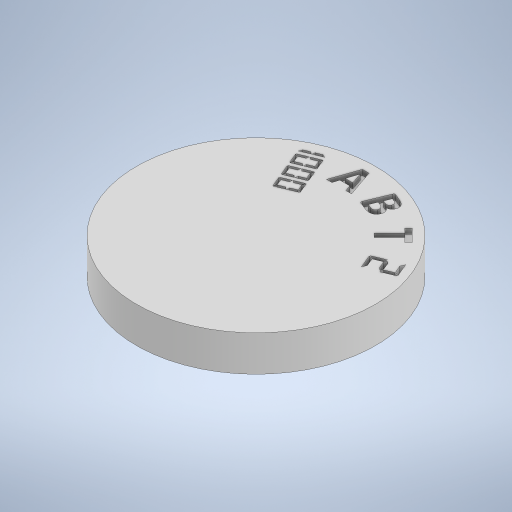
# Autodesk Inventor part: rot_th
Saved by Autodesk Inventor 2023 (Build 270158000, 158)
## iProperties
Created: 2023-05-20
Part Number: rot_th
Material: 常规
Document SubType Name: Modeling
Designer: LiuZeshu
Density: 1 g/cm^3
Appearance: 默认
Author: LiuZeshu
Autodesk Inventor part; units mm, degrees
ref_plane "YZ Plane" through (0, 0, 0) normal (1, 0, 0) x (0, 1, 0)
ref_plane "XZ Plane" through (0, 0, 0) normal (0, 1, 0) x (-1, 0, 0)
ref_plane "XY Plane" through (0, 0, 0) normal (0, 0, 1) x (1, 0, 0)
sketch "草图1" plane through (0, 0, 0) normal (0, 1, 0) x (-1, 0, 0)
  arc A0 (1.3748, -0.6) -> (-1.3748, -0.6) centre (0, 0) ccw
  line L0 (1.3748, -0.6) -> (-1.3748, -0.6)
  circle A1 centre (0, 0) radius 9
  dimension "d0" = 3
  dimension "d1" = 2.1
  dimension "d2" = 18
  constraints: 2 centre point, 2 coincident, 2 end point, 2 point on circle, 1 horizontal
  measures "d0" diameter of A0
  measures "d2" diameter of A1
extrude "拉伸1" add sketch "草图1" along normal blind 2.3
sketch "草图2" plane through (0, 2.3, 0) normal (0, 1, 0) x (1, 0, 0)
  circle A0 centre (0, 0) radius 9
  dimension "d7" = 18
  constraints: 1 centre point, 1 coincident
  measures "d7" diameter of A0
extrude "拉伸2" add sketch "草图2" along normal blind 0.4
sketch "草图3" plane through (0, 2.7, 0) normal (0, 1, 0) x (1, 0, 0)
  line L0 (0, 0) -> (0, 10.4823)
  line L1 (-0.7481, 7.9877) -> (0.7481, 7.9877) construction
  line L2 (0.7481, 7.9877) -> (0.7481, 6.3) construction
  line L3 (0.7481, 6.3) -> (-0.7481, 6.3) construction
  line L4 (-0.7481, 6.3) -> (-0.7481, 7.9877) construction
  line L5 (0, 0) -> (-4.0114, 9.6844)
  line L6 (0, 0) -> (-7.4121, 7.4121)
  line L7 (0, 0) -> (-9.6844, 4.0114)
  line L8 (0, 0) -> (-10.4823, 0)
  line L9 (0, 0) -> (-9.6844, -4.0114)
  line L10 (0, 0) -> (-7.4121, -7.4121)
  line L11 (0, 0) -> (-4.0114, -9.6844)
  line L12 (0, 0) -> (0, -10.4823)
  line L13 (0, 0) -> (4.0114, -9.6844)
  line L14 (0, 0) -> (7.4121, -7.4121)
  line L15 (0, 0) -> (9.6844, -4.0114)
  line L16 (0, 0) -> (10.4823, 0)
  line L17 (0, 0) -> (9.6844, 4.0114)
  line L18 (0, 0) -> (7.4121, 7.4121)
  line L19 (0, 0) -> (4.0114, 9.6844)
  line L20 (2.0839, 8.406) -> (4.4704, 7.4175) construction
  line L21 (4.4704, 7.4175) -> (3.6042, 5.3262) construction
  line L22 (3.6042, 5.3262) -> (1.2176, 6.3147) construction
  line L23 (1.2176, 6.3147) -> (2.0839, 8.406) construction
  line L24 (3.5415, 5.3681) -> (4.5678, 6.3944) construction
  line L25 (4.5678, 6.3944) -> (6.3944, 4.5678) construction
  line L26 (6.3944, 4.5678) -> (5.3681, 3.5415) construction
  line L27 (5.3681, 3.5415) -> (3.5415, 5.3681) construction
  line L28 (5.3262, 3.6042) -> (6.9301, 4.2685) construction
  line L29 (6.9301, 4.2685) -> (7.9186, 1.882) construction
  line L30 (7.9186, 1.882) -> (6.3147, 1.2176) construction
  line L31 (6.3147, 1.2176) -> (5.3262, 3.6042) construction
  line L32 (-4.0975, 7.4844) -> (-2.3949, 8.1897) construction
  line L33 (-2.3949, 8.1897) -> (-1.0621, 4.972) construction
  line L34 (-1.0621, 4.972) -> (-2.7647, 4.2668) construction
  line L35 (-2.7647, 4.2668) -> (-4.0975, 7.4844) construction
  line L36 (0.9024, 6.3013) -> (0.4624, 6.3013)
  line L37 (0.4624, 6.3013) -> (0.3119, 6.7554)
  line L38 (0.3119, 6.7554) -> (-0.4394, 6.7554)
  line L39 (-0.4394, 6.7554) -> (-0.5848, 6.3013)
  line L40 (-0.5848, 6.3013) -> (-0.9917, 6.3013)
  line L41 (-0.9917, 6.3013) -> (-0.2953, 8.3089)
  line L42 (-0.2953, 8.3089) -> (0.2034, 8.3089)
  line L43 (0.2034, 8.3089) -> (0.9024, 6.3013)
  line L44 (-0.0657, 7.9173) -> (-0.067, 7.9173)
  line L45 (-0.067, 7.9173) -> (-0.3501, 7.0679)
  line L46 (-0.3501, 7.0679) -> (0.2175, 7.0679)
  line L47 (0.2175, 7.0679) -> (-0.0657, 7.9173)
  spline S0 degree 2 poles (3.3024, 6.1028) (3.2614, 6.0038) (3.1408, 5.866) (2.9946, 5.783) (2.825, 5.7469) (2.6413, 5.7568) (2.4486, 5.8048) (2.3378, 5.8507) knots 0 0 0 1 2 3 4 5 6 6 6
  line L48 (2.3378, 5.8507) -> (1.8464, 6.0542)
  spline S1 degree 2 poles (1.8464, 6.0542) (1.7993, 6.0738) (1.7586, 6.1555) (1.785, 6.2192) knots 0 0 0 1 2 2 2
  line L49 (1.785, 6.2192) -> (2.4552, 7.8371)
  spline S2 degree 2 poles (2.4552, 7.8371) (2.481, 7.8996) (2.5676, 7.9286) (2.6147, 7.9091) knots 0 0 0 1 2 2 2
  line L50 (2.6147, 7.9091) -> (3.079, 7.7168)
  spline S3 degree 2 poles (3.079, 7.7168) (3.2487, 7.6465) (3.461, 7.4923) (3.5736, 7.3076) (3.5852, 7.0957) (3.535, 6.9743) knots 0 0 0 1 2 3 4 4 4
  spline S4 degree 2 poles (3.535, 6.9743) (3.5071, 6.9071) (3.4242, 6.8034) (3.3181, 6.7341) (3.191, 6.6971) (3.1204, 6.7001) knots 0 0 0 1 2 3 4 4 4
  spline S5 degree 2 poles (3.1204, 6.7001) (3.1935, 6.6532) (3.2957, 6.5267) (3.3483, 6.3737) (3.3414, 6.1971) (3.3024, 6.1028) knots 0 0 0 1 2 3 4 4 4
  spline S6 degree 2 poles (2.9081, 6.2509) (2.935, 6.3157) (2.9334, 6.4352) (2.8797, 6.5388) (2.7668, 6.6298) (2.6643, 6.6722) knots 0 0 0 1 2 3 4 4 4
  line L51 (2.6643, 6.6722) -> (2.4416, 6.7645)
  line L52 (2.4416, 6.7645) -> (2.2229, 6.2366)
  line L53 (2.2229, 6.2366) -> (2.494, 6.1243)
  spline S7 degree 2 poles (2.494, 6.1243) (2.5729, 6.0916) (2.6933, 6.079) (2.798, 6.1116) (2.8828, 6.1897) (2.9081, 6.2509) knots 0 0 0 1 2 3 4 4 4
  spline S8 degree 2 poles (3.1417, 7.0847) (3.1651, 7.1413) (3.1675, 7.2438) (3.1224, 7.3315) (3.0314, 7.4051) (2.9442, 7.4413) knots 0 0 0 1 2 3 4 4 4
  line L54 (2.9442, 7.4413) -> (2.7545, 7.5198)
  line L55 (2.7545, 7.5198) -> (2.5553, 7.0391)
  line L56 (2.5553, 7.0391) -> (2.7651, 6.9522)
  spline S9 degree 2 poles (2.7651, 6.9522) (2.8464, 6.9185) (2.9603, 6.9169) (3.0518, 6.9577) (3.1207, 7.0341) (3.1417, 7.0847) knots 0 0 0 1 2 3 4 4 4
  line L57 (6.0737, 5.1447) -> (5.7508, 5.4676)
  line L58 (5.7508, 5.4676) -> (4.5973, 4.3141)
  line L59 (4.5973, 4.3141) -> (4.3087, 4.6009)
  line L60 (4.3087, 4.6009) -> (5.4613, 5.7535)
  line L61 (5.4613, 5.7535) -> (5.1402, 6.0746)
  line L62 (5.1402, 6.0746) -> (5.4108, 6.3452)
  line L63 (5.4108, 6.3452) -> (6.3425, 5.4135)
  line L64 (6.3425, 5.4135) -> (6.0737, 5.1447)
  line L65 (-3.2171, 7.3838) -> (-3.9038, 7.0994)
  line L66 (-3.9038, 7.0994) -> (-3.8055, 7.3369)
  line L67 (-3.8055, 7.3369) -> (-3.3848, 7.5111)
  line L68 (-3.3848, 7.5111) -> (-3.2171, 7.3838)
  line L69 (-2.5012, 7.6804) -> (-3.1879, 7.3959)
  line L70 (-3.1879, 7.3959) -> (-3.1594, 7.6045)
  line L71 (-3.1594, 7.6045) -> (-2.7387, 7.7787)
  line L72 (-2.7387, 7.7787) -> (-2.5012, 7.6804)
  line L73 (-3.4977, 6.0365) -> (-3.8122, 6.7957)
  line L74 (-3.8122, 6.7957) -> (-3.5747, 6.6973)
  line L75 (-3.5747, 6.6973) -> (-3.3994, 6.2739)
  line L76 (-3.3994, 6.2739) -> (-3.4977, 6.0365)
  line L77 (-2.0368, 6.6416) -> (-2.2743, 6.74)
  line L78 (-2.2743, 6.74) -> (-2.4496, 7.1633)
  line L79 (-2.4496, 7.1633) -> (-2.3512, 7.4008)
  line L80 (-2.3512, 7.4008) -> (-2.0368, 6.6416)
  line L81 (-3.0792, 7.1334) -> (-2.3925, 7.4179)
  line L82 (-2.3925, 7.4179) -> (-2.4909, 7.1804)
  line L83 (-2.4909, 7.1804) -> (-2.9116, 7.0061)
  line L84 (-2.9116, 7.0061) -> (-3.0792, 7.1334)
  line L85 (-2.7694, 6.3029) -> (-3.4561, 6.0185)
  line L86 (-3.4561, 6.0185) -> (-3.3577, 6.256)
  line L87 (-3.3577, 6.256) -> (-2.937, 6.4302)
  line L88 (-2.937, 6.4302) -> (-2.7694, 6.3029)
  line L89 (-3.7951, 6.8369) -> (-3.1084, 7.1214)
  line L90 (-3.1084, 7.1214) -> (-3.1369, 6.9128)
  line L91 (-3.1369, 6.9128) -> (-3.5576, 6.7385)
  line L92 (-3.5576, 6.7385) -> (-3.7951, 6.8369)
  line L93 (-2.0535, 6.5995) -> (-2.7402, 6.315)
  line L94 (-2.7402, 6.315) -> (-2.7117, 6.5236)
  line L95 (-2.7117, 6.5236) -> (-2.291, 6.6978)
  line L96 (-2.291, 6.6978) -> (-2.0535, 6.5995)
  line L97 (-1.5891, 5.5607) -> (-1.8265, 5.6591)
  line L98 (-1.8265, 5.6591) -> (-2.0019, 6.0824)
  line L99 (-2.0019, 6.0824) -> (-1.9035, 6.3199)
  line L100 (-1.9035, 6.3199) -> (-1.5891, 5.5607)
  line L101 (-3.05, 4.9556) -> (-3.3645, 5.7148)
  line L102 (-3.3645, 5.7148) -> (-3.127, 5.6164)
  line L103 (-3.127, 5.6164) -> (-2.9516, 5.193)
  line L104 (-2.9516, 5.193) -> (-3.05, 4.9556)
  line L105 (-2.6315, 6.0525) -> (-1.9448, 6.337)
  line L106 (-1.9448, 6.337) -> (-2.0431, 6.0995)
  line L107 (-2.0431, 6.0995) -> (-2.4638, 5.9252)
  line L108 (-2.4638, 5.9252) -> (-2.6315, 6.0525)
  line L109 (-1.6058, 5.5186) -> (-2.2925, 5.2341)
  line L110 (-2.2925, 5.2341) -> (-2.2639, 5.4427)
  line L111 (-2.2639, 5.4427) -> (-1.8433, 5.6169)
  line L112 (-1.8433, 5.6169) -> (-1.6058, 5.5186)
  line L113 (-2.3217, 5.222) -> (-3.0084, 4.9376)
  line L114 (-3.0084, 4.9376) -> (-2.91, 5.1751)
  line L115 (-2.91, 5.1751) -> (-2.4893, 5.3493)
  line L116 (-2.4893, 5.3493) -> (-2.3217, 5.222)
  line L117 (-3.3474, 5.756) -> (-2.6607, 6.0405)
  line L118 (-2.6607, 6.0405) -> (-2.6892, 5.8319)
  line L119 (-2.6892, 5.8319) -> (-3.1099, 5.6576)
  line L120 (-3.1099, 5.6576) -> (-3.3474, 5.756)
  line L121 (-1.1413, 4.4798) -> (-1.3788, 4.5782)
  line L122 (-1.3788, 4.5782) -> (-1.5542, 5.0015)
  line L123 (-1.5542, 5.0015) -> (-1.4558, 5.239)
  line L124 (-1.4558, 5.239) -> (-1.1413, 4.4798)
  line L125 (-2.6023, 3.8747) -> (-2.9167, 4.6339)
  line L126 (-2.9167, 4.6339) -> (-2.6793, 4.5355)
  line L127 (-2.6793, 4.5355) -> (-2.5039, 4.1121)
  line L128 (-2.5039, 4.1121) -> (-2.6023, 3.8747)
  line L129 (-2.1838, 4.9716) -> (-1.497, 5.2561)
  line L130 (-1.497, 5.2561) -> (-1.5954, 5.0186)
  line L131 (-1.5954, 5.0186) -> (-2.0161, 4.8443)
  line L132 (-2.0161, 4.8443) -> (-2.1838, 4.9716)
  line L133 (-1.8739, 4.1411) -> (-2.5607, 3.8567)
  line L134 (-2.5607, 3.8567) -> (-2.4623, 4.0942)
  line L135 (-2.4623, 4.0942) -> (-2.0416, 4.2684)
  line L136 (-2.0416, 4.2684) -> (-1.8739, 4.1411)
  line L137 (-2.8997, 4.6751) -> (-2.2129, 4.9595)
  line L138 (-2.2129, 4.9595) -> (-2.2415, 4.751)
  line L139 (-2.2415, 4.751) -> (-2.6622, 4.5767)
  line L140 (-2.6622, 4.5767) -> (-2.8997, 4.6751)
  line L141 (-1.158, 4.4377) -> (-1.8448, 4.1532)
  line L142 (-1.8448, 4.1532) -> (-1.8162, 4.3618)
  line L143 (-1.8162, 4.3618) -> (-1.3955, 4.536)
  line L144 (-1.3955, 4.536) -> (-1.158, 4.4377)
  line L145 (6.0301, 1.9048) -> (5.6108, 2.917)
  line L146 (5.6108, 2.917) -> (5.9274, 2.7859)
  line L147 (5.9274, 2.7859) -> (6.1612, 2.2214)
  line L148 (6.1612, 2.2214) -> (6.0301, 1.9048)
  line L149 (7.978, 2.7116) -> (7.6614, 2.8428)
  line L150 (7.6614, 2.8428) -> (7.4276, 3.4073)
  line L151 (7.4276, 3.4073) -> (7.5587, 3.7239)
  line L152 (7.5587, 3.7239) -> (7.978, 2.7116)
  line L153 (6.6089, 3.2573) -> (6.8026, 3.1263)
  line L154 (6.8026, 3.1263) -> (7.0188, 2.6042)
  line L155 (7.0188, 2.6042) -> (6.9749, 2.3735)
  line L156 (6.9749, 2.3735) -> (6.7772, 2.5042)
  line L157 (6.7772, 2.5042) -> (6.561, 3.0262)
  line L158 (6.561, 3.0262) -> (6.6089, 3.2573)
  line L159 (7.9557, 2.6555) -> (7.0401, 2.2762)
  line L160 (7.0401, 2.2762) -> (7.0782, 2.5543)
  line L161 (7.0782, 2.5543) -> (7.6391, 2.7866)
  line L162 (7.6391, 2.7866) -> (7.9557, 2.6555)
  line L163 (5.6336, 2.972) -> (6.5492, 3.3513)
  line L164 (6.5492, 3.3513) -> (6.5111, 3.0732)
  line L165 (6.5111, 3.0732) -> (5.9502, 2.8409)
  line L166 (5.9502, 2.8409) -> (5.6336, 2.972)
  point P0 (0, 7.9877)
  point P1 (0, 7.9877)
  point P2 (-3.0568, 7.3797)
  point P3 (-3.0568, 7.3797)
  point P4 (-5.6481, 5.6481)
  point P5 (-5.6481, 5.6481)
  point P6 (-7.3797, 3.0568)
  point P7 (-7.3797, 3.0568)
  point P8 (-7.9877, 0)
  point P9 (-7.9877, 0)
  point P10 (-7.3797, -3.0568)
  point P11 (-7.3797, -3.0568)
  point P12 (-5.6481, -5.6481)
  point P13 (-5.6481, -5.6481)
  point P14 (-3.0568, -7.3797)
  point P15 (-3.0568, -7.3797)
  point P16 (0, -7.9877)
  point P17 (0, -7.9877)
  point P18 (3.0568, -7.3797)
  point P19 (3.0568, -7.3797)
  point P20 (5.6481, -5.6481)
  point P21 (5.6481, -5.6481)
  point P22 (7.3797, -3.0568)
  point P23 (7.3797, -3.0568)
  point P24 (7.9877, 0)
  point P25 (7.9877, 0)
  point P26 (7.3797, 3.0568)
  point P27 (7.3797, 3.0568)
  point P28 (5.6481, 5.6481)
  point P29 (5.6481, 5.6481)
  point P30 (3.0568, 7.3797)
  point P31 (3.0568, 7.3797)
  point P32 (1.625, 8.5961)
  point P33 (3.2772, 7.9117)
  point P34 (2.6779, 8.2844)
  point P35 (5.4811, 5.4811)
  point P36 (5.427, 7.8973)
  point P37 (7.4243, 3.0753)
  point P38 (-0.8523, 4.4654)
  point P39 (-1.7285, 6.5808)
  point P40 (-3.2462, 7.837)
  dimension "d17" = 360
  dimension "d19" = 6.3
  dimension "d20" = 6.3
  dimension "d21" = 6.3
  dimension "d22" = 6.3
  dimension "d23" = 5
  constraints: 32 end point, 25 point on line, 7 midpoint, 5 perpendicular, 3 coincident, 1 vertical, 89 other
  measures "d19" distance from line of L0.start L3
  measures "d20" distance from line of L0.start L22
  measures "d21" distance from line of L0.start L27
  measures "d22" distance from line of L0.start L31
  measures "d23" distance from line of L0.start L34
extrude "拉伸3" cut sketch "草图3" against normal blind 0.4 contours L38 L39 L40 L41 L42 L0 L47 L45 L46 | L0 L46 L47 L42 L43 L36 L37 L38 | L69 L70 L71 L5 | L5 L71 L72 L69 | L83 L84 L81 L5 | L5 L81 L82 L83 | L93 L94 L95 L5 | L5 L95 L96 L93 | L107 L108 L105 L5 | L5 L105 L106 L107 | L109 L110 L111 L5 | L5 L111 L112 L109 | L131 L132 L129 L5 | L5 L129 L130 L131 | L141 L142 L143 L5 | L5 L143 L144 L141 | L150 L151 L152 L17 | L17 L152 L149 L150 | L157 L158 L153 L154 L17 | L17 L154 L155 L156 L157 | L145 L146 L147 L17 | L17 L147 L148 L145 | L59 L60 L61 L62 L63 L18 | L18 L63 L64 L57 L58 L59 | S0 L48 S1 L49 S2 L50 S3 L19 S8 L54 L55 L56 S9 S6 L51 L52 L53 S7 | L19 S7 S6 S9 S8 S3 S4 S5 S0 | L65 L66 L67 L68 | L73 L74 L75 L76 | L77 L78 L79 L80 | L85 L86 L87 L88 | L89 L90 L91 L92 | L97 L98 L99 L100 | L101 L102 L103 L104 | L113 L114 L115 L116 | L117 L118 L119 L120 | L121 L122 L123 L124 | L125 L126 L127 L128 | L133 L134 L135 L136 | L137 L138 L139 L140 | L159 L160 L161 L162 | L163 L164 L165 L166
